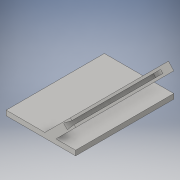
# Autodesk Inventor part: proto_1_base
Saved by Autodesk Inventor 2016 (Build 200138000, 138)
## iProperties
Created: 2017-07-19
Part Number: proto_1_base
Material: Generic
Document SubType Name: Modeling
Designer: Logan
Density: 1 g/cm^3
Appearance: Default
Author: Logan
Autodesk Inventor part; units mm, degrees
ref_plane "YZ Plane" through (0, 0, 0) normal (1, 0, 0) x (0, 1, 0)
ref_plane "XZ Plane" through (0, 0, 0) normal (0, 1, 0) x (-1, 0, 0)
ref_plane "XY Plane" through (0, 0, 0) normal (0, 0, 1) x (1, 0, 0)
sketch "Sketch1" plane through (0, 0, 0) normal (0, 0, 1) x (1, 0, 0)
  line L0 (44.9013, -57.6013) -> (44.9013, -83.0013) construction
  line L1 (-44.9013, -83.0013) -> (44.9013, -83.0013)
  line L2 (-44.9013, -83.0013) -> (-44.9013, -89.3513)
  line L3 (44.9013, -83.0013) -> (44.9013, -89.3513)
  line L4 (44.9013, -83.0013) -> (51.2513, -83.0013) construction
  line L5 (-44.9013, -89.3513) -> (44.9013, -89.3513)
  line L6 (44.9013, -57.6013) -> (19.5013, -83.0013)
  line L7 (44.9013, -57.6013) -> (80.8223, -57.6013) construction
  line L8 (44.9013, -57.6013) -> (37.9664, -50.1761) construction
  line L9 (37.9664, -50.1761) -> (5.1412, -83.0013)
  line L10 (37.9664, -50.1761) -> (84.3883, -50.1761) construction
  line L11 (37.9664, -50.1761) -> (44.9013, -57.6013)
  dimension "d4" = 25.4
  dimension "d7" = 6.35
  dimension "d8" = 90
  dimension "d9" = 135
  dimension "d10" = 10.16
  dimension "d11" = 135
  constraints: 24 end point, 4 equal length, 4 horizontal, 2 point on line, 1 collinear, 1 perpendicular
  measures "d4" distance of L0.start L0.end
  measures "d7" distance of L1.start L2.end
  measures "d8" angle of L3 L4
  measures "d9" angle of L6 L7
  measures "d10" distance of L0.start L8.end
  measures "d11" angle of L9 L10
extrude "Extrusion1" add sketch "Sketch1" against normal blind 127
sketch "Sketch5" plane through (0, 0, 0) normal (0, 0, 1) x (1, 0, 0)
  line L0 (39.9602, -52.3108) -> (42.9075, -55.4665)
  line L1 (44.9013, -57.6013) -> (37.9664, -50.1761) projected
  line L2 (29.4406, -60.398) -> (34.1216, -65.41)
  line L3 (41.4339, -53.8887) -> (31.7811, -62.904) construction
  line L4 (29.4406, -60.398) -> (39.9602, -52.3108)
  line L5 (34.1216, -65.41) -> (42.9075, -55.4665)
  point P0 (0, 0)
  dimension "d28" = 4.318
  dimension "d29" = 6.858
  dimension "d30" = 13.208
  constraints: 10 end point, 4 midpoint, 1 collinear, 1 parallel, 1 perpendicular
  measures "d28" distance of L0.start L0.end
  measures "d29" distance of L2.start L2.end
  measures "d30" distance of L3.start L3.end
extrude "Extrusion5" cut sketch "Sketch5" against normal blind 114.808
body "Solid1"
